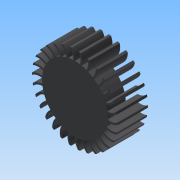
# Autodesk Inventor part: 4020
Saved by Autodesk Inventor 2017 (Build 210142000, 142)
## iProperties
Part Number: 4020
Material: Типовые
Document SubType Name: Modeling
Designer: Max
Mass: 5.03449 g
Surface Area: 54.2386 cm^2
Volume: 5.03449 cm^3
Density: 1 g/cm^3
Appearance: Серый
Author: Max
Autodesk Inventor part; units mm, degrees
ref_plane "YZ Plane" through (0, 0, 0) normal (1, 0, 0) x (0, 1, 0)
ref_plane "XZ Plane" through (0, 0, 0) normal (0, 1, 0) x (-1, 0, 0)
ref_plane "XY Plane" through (0, 0, 0) normal (0, 0, 1) x (1, 0, 0)
sketch "Эскиз1" plane through (0, 0, 0) normal (0, 1, 0) x (-1, 0, 0)
  line L0 (0, 0) -> (0, 30)
  line L1 (0, 30) -> (20.3, 30)
  line L2 (-62.0243, 51.3971) -> (67.3361, 51.3971) construction
  line L3 (67.3361, 51.3971) -> (67.3361, -36.2164) construction
  line L4 (67.3361, -36.2164) -> (-62.0243, -36.2164) construction
  line L5 (-62.0243, -36.2164) -> (-62.0243, 51.3971) construction
  line L6 (20.3, 30) -> (20.3, -25.8683) construction
  line L7 (0, 8.5) -> (47.9124, 8.5) construction
  line L8 (20.3, 30) -> (64.5237, 30) construction
  circle A0 centre (37.8, 27.3) radius 3
  circle A1 centre (37.8, 27.3) radius 1.75
  line L9 (37.8, 27.3) -> (37.8, -7.8) construction
  circle A2 centre (37.8, -7.8) radius 1.75
  circle A3 centre (37.8, -7.8) radius 3
  line L10 (37.8, -7.8) -> (2.8, -7.8) construction
  circle A4 centre (2.8, -7.8) radius 1.75
  circle A5 centre (2.8, -7.8) radius 3
  line L11 (2.8, -7.8) -> (37.8, 27.3) construction
  line L12 (0, 30) -> (40.5, 30) construction
  line L13 (40.5, 30) -> (40.5, -10.5) construction
  line L14 (40.5, -10.5) -> (0, -10.5) construction
  line L15 (0, -10.5) -> (0, 30) construction
  line L16 (0, 0) -> (10.5411, -7.8)
  arc A6 (10.5411, -7.8) -> (30.3802, -7.8) centre (20.4606, 9.7079) ccw
  arc A7 (30.3802, -7.8) -> (40.5, 8.5) centre (20.5113, 9.6185) ccw
  arc A8 (40.5, 8.5) -> (20.3, 30) centre (20.315, 9.7748) ccw
  arc A9 (1.0609, -4.676) -> (0, 0) centre (-2.1861, -2.9543) ccw
  line L17 (0.1496, -6.3946) -> (1.0609, -4.676)
  line L18 (4.7164, -10.1081) -> (7.2118, -8.0362)
  arc A10 (10.5411, -7.8) -> (7.2118, -8.0362) centre (9.0411, -10.2394) ccw
  arc A11 (35.6753, -9.9179) -> (30.3802, -7.8) centre (30.5679, -15.009) ccw
  arc A12 (38.0693, 0) -> (39.868, -5.6267) centre (44.1082, -1.1704) ccw
  arc A13 (29.7654, 27.6564) -> (35.6321, 29.3737) centre (31.2088, 33.6047) ccw
  arc A14 (39.8419, 25.1021) -> (38.1561, 19.3013) centre (43.8447, 20.7935) ccw
  circle A15 centre (20.3, 8.5) radius 14
  arc A16 (30.1091, -7.3215) -> (39.951, 8.5327) centre (20.5113, 9.6185) ccw
  arc A17 (39.951, 8.5327) -> (20.315, 29.45) centre (20.315, 9.7748) ccw
  line L19 (20.315, 29.45) -> (0, 29.45)
  arc A18 (10.8122, -7.3215) -> (30.1091, -7.3215) centre (20.4606, 9.7079) ccw
  line L20 (10.8122, -7.3215) -> (3.3428, 1.6745)
  line L21 (3.3428, 1.6745) -> (0, 1.5217)
  line L22 (0, 1.5217) -> (0, 0)
  line L23 (0, 29.45) -> (0, 30)
  line L24 (0, 29.45) -> (0, 30)
  circle A19 centre (20.3, 8.5) radius 11.5
  circle A20 centre (20.3, 8.5) radius 17
  dimension "d0" = 30
  dimension "d1" = 20.3
  dimension "d2" = 3.5
  dimension "d3" = 17.5
  dimension "d4" = 18.8
  dimension "d5" = 3.5
  dimension "d6" = 16.3
  dimension "d7" = 17.5
  dimension "d8" = 17.5
  dimension "d9" = 3.5
  dimension "d10" = 40.5
  dimension "d11" = 40.5
  dimension "d12" = 21.5
  dimension "d13" = 6
  dimension "d14" = 6
  dimension "d15" = 6
  dimension "d16" = 126.5
  dimension "d17" = 20.2252
  dimension "d18" = 20.0199
  dimension "d19" = 20.1228
  dimension "d20" = 3.6082
  dimension "d21" = 7.2115
  dimension "d22" = 2.8637
  dimension "d23" = 39.703
  dimension "d24" = 0.9113
  dimension "d25" = 6.1513
  dimension "d26" = 5.881
  dimension "d27" = 6.121
  dimension "d28" = 5.8008
  dimension "d29" = 5.8667
  dimension "d30" = 28
  dimension "d31" = 0.55
  dimension "d32" = 0.55
  dimension "d35" = 23
  dimension "d36" = 34
  constraints: 42 end point, 33 point on circle, 21 centre point, 10 tangent, 9 point on line, 7 coincident, 3 collinear, 3 horizontal, 3 perpendicular, 3 vertical, 2 parallel, 3 other
  measures "d0" distance of L0.start L0.end
  measures "d1" distance of L0.end L1.end
  measures "d2" diameter of A1
  measures "d3" distance from line of A0.centre L6
  measures "d4" distance from line of L7 A0.centre
  measures "d5" diameter of A2
  measures "d6" distance from line of L9.end L7
  measures "d7" distance from line of L9.end L6
  measures "d8" distance from line of L6 L10.end
  measures "d9" diameter of A4
  measures "d10" distance of L13.end L14.end
  measures "d11" distance of L12.end L13.end
  measures "d12" distance between parallel lines of L7 L8
  measures "d13" diameter of A0
  measures "d14" diameter of A3
  measures "d15" diameter of A5
  measures "d16" angle of L15 L16
  measures "d17" radius of A8
  measures "d18" radius of A7
  measures "d19" radius of A6
  measures "d20" distance from line of L13 A12.centre
  measures "d21" radius of A11
  measures "d22" radius of A10
  measures "d23" angle of L14 L18
  measures "d24" horizontal distance of L17.start L17.end
  measures "d25" radius of A12
  measures "d26" radius of A14
  measures "d27" radius of A13
  measures "d28" vertical distance of A14.end A0.end
  measures "d29" horizontal distance of A0.start A13.start
  measures "d30" diameter of A15
  measures "d31" radial gap between concentric circles of A7 A16
  measures "d32" radial gap between concentric circles of A6 A18
  measures "d35" diameter of A19
  measures "d36" diameter of A20
extrude "Выдавливание1" add sketch "Эскиз1" along normal blind 12 contours A15 | A19 | A20
sketch "Эскиз2" plane through (-20.3, 12, 8.5) normal (0, 1, 0) x (1, 0, 0)
  circle A0 centre (0, 0) radius 11.5
  circle A1 centre (0, 0) radius 13
  circle A2 centre (0, 0) radius 17 projected
  arc A3 (1.2, 16.9576) -> (0, 13) centre (5.6832, 13.4375) ccw
  arc A4 (2.0528, 16.8756) -> (0.7041, 12.9809) centre (5.6832, 13.4375) ccw
  line L0 (0, 0) -> (0, 22.7332) construction
  point P0 (20.3, 8.5)
  dimension "d40" = 23
  dimension "d41" = 26
  dimension "d42" = 0.7
  dimension "d43" = 1.2
  dimension "d44" = 5
  constraints: 8 point on circle, 4 centre point, 3 coincident, 2 end point, 1 point on line, 1 vertical
  measures "d40" diameter of A0
  measures "d41" diameter of A1
  measures "d42" radial gap between concentric circles of A4 A3
  measures "d43" distance from line of L0 A2.start
  measures "d44" radius of A4
extrude "Выдавливание2" cut sketch "Эскиз2" against normal blind 12 contours A1 A4 A2 A3 | A1 A3 A2 A4
extrude "Выдавливание3" add sketch "Эскиз2" against normal blind 12 contours A1 A3 A2 A4 picked at (0.2619, 13.8155)
pattern_circular "Круговой массив2" count 30 over 360 about axis through (-20.3, 12, 8.5) along (0, -1, 0) of "Выдавливание3"
sketch "Эскиз3" plane through (0, 12, 0) normal (0, 1, 0) x (1, 0, 0)
  arc A0 (-20.3, 4.5) -> (-22.3102, 4.3436) centre (-20.3, -8.5) ccw projected
  arc A1 (-21.8007, 8.4336) -> (-22.3102, 4.3436) centre (-17.5348, 5.8255) ccw projected
  arc A2 (-21.8007, 8.4336) -> (-22.6519, 8.3365) centre (-20.3, -8.5) ccw projected
  arc A3 (-22.6519, 8.3365) -> (-23.0029, 4.2159) centre (-17.5348, 5.8255) ccw projected
  arc A4 (-23.0029, 4.2159) -> (-24.9366, 3.645) centre (-20.3, -8.5) ccw projected
  arc A5 (-25.2886, 7.7516) -> (-24.9366, 3.645) centre (-20.5737, 6.0873) ccw projected
  arc A6 (-25.2886, 7.7516) -> (-26.101, 7.4796) centre (-20.3, -8.5) ccw projected
  arc A7 (-26.101, 7.4796) -> (-25.5876, 3.3761) centre (-20.5737, 6.0873) ccw projected
  arc A8 (-25.5876, 3.3761) -> (-27.3604, 2.4156) centre (-20.3, -8.5) ccw projected
  arc A9 (-28.5585, 6.3593) -> (-27.3604, 2.4156) centre (-23.6006, 5.7117) ccw projected
  arc A10 (-28.5585, 6.3593) -> (-29.2966, 5.9243) centre (-20.3, -8.5) ccw projected
  arc A11 (-29.2966, 5.9243) -> (-27.9412, 2.0172) centre (-23.6006, 5.7117) ccw projected
  arc A12 (-27.9412, 2.0172) -> (-29.4756, 0.7092) centre (-20.3, -8.5) ccw projected
  arc A13 (-31.4674, 4.3175) -> (-29.4756, 0.7092) centre (-26.4832, 4.7149) ccw projected
  arc A14 (-31.4674, 4.3175) -> (-32.099, 3.7386) centre (-20.3, -8.5) ccw projected
  arc A15 (-32.099, 3.7386) -> (-29.9609, 0.1987) centre (-26.4832, 4.7149) ccw projected
  arc A16 (-29.9609, 0.1987) -> (-31.1898, -1.3998) centre (-20.3, -8.5) ccw projected
  arc A17 (-33.8883, 1.7156) -> (-31.1898, -1.3998) centre (-29.0956, 3.1405) ccw projected
  arc A18 (-33.8883, 1.7156) -> (-34.3857, 1.018) centre (-20.3, -8.5) ccw projected
  arc A19 (-34.3857, 1.018) -> (-31.5583, -2) centre (-29.0956, 3.1405) ccw projected
  arc A20 (-31.5583, -2) -> (-32.428, -3.8191) centre (-20.3, -8.5) ccw projected
  arc A21 (-35.7153, -1.3328) -> (-32.428, -3.8191) centre (-31.3236, 1.0574) ccw projected
  arc A22 (-35.7153, -1.3328) -> (-36.0568, -2.1185) centre (-20.3, -8.5) ccw projected
  arc A23 (-36.0568, -2.1185) -> (-32.6637, -4.4828) centre (-31.3236, 1.0574) ccw projected
  arc A24 (-32.6637, -4.4828) -> (-33.1362, -6.4429) centre (-20.3, -8.5) ccw projected
  arc A25 (-36.8686, -4.6944) -> (-33.1362, -6.4429) centre (-33.0698, -1.4433) ccw projected
  arc A26 (-36.8686, -4.6944) -> (-37.0393, -5.534) centre (-20.3, -8.5) ccw projected
  arc A27 (-37.0393, -5.534) -> (-33.2288, -7.1411) centre (-33.0698, -1.4433) ccw projected
  arc A28 (-33.2288, -7.1411) -> (-33.2834, -9.1567) centre (-20.3, -8.5) ccw projected
  arc A29 (-37.2977, -8.2224) -> (-33.2834, -9.1567) centre (-34.2579, -4.2525) ccw projected
  arc A30 (-37.2977, -8.2224) -> (-37.2901, -9.0791) centre (-20.3, -8.5) ccw projected
  arc A31 (-37.2901, -9.0791) -> (-33.2288, -9.8589) centre (-34.2579, -4.2525) ccw projected
  arc A32 (-33.2288, -9.8589) -> (-32.8632, -11.8417) centre (-20.3, -8.5) ccw projected
  arc A33 (-36.984, -11.7625) -> (-32.8632, -11.8417) centre (-34.836, -7.2474) ccw projected
  arc A34 (-36.984, -11.7625) -> (-36.7985, -12.5989) centre (-20.3, -8.5) ccw projected
  arc A35 (-36.7985, -12.5989) -> (-32.6637, -12.5172) centre (-34.836, -7.2474) ccw projected
  arc A36 (-32.6637, -12.5172) -> (-31.8938, -14.3807) centre (-20.3, -8.5) ccw projected
  arc A37 (-35.9411, -15.16) -> (-31.8938, -14.3807) centre (-34.7788, -10.297) ccw projected
  arc A38 (-35.9411, -15.16) -> (-35.5857, -15.9396) centre (-20.3, -8.5) ccw projected
  arc A39 (-35.5857, -15.9396) -> (-31.5583, -15) centre (-34.7788, -10.297) ccw projected
  arc A40 (-31.5583, -15) -> (-30.4178, -16.6627) centre (-20.3, -8.5) ccw projected
  arc A41 (-34.2146, -18.2664) -> (-30.4178, -16.6627) centre (-34.0888, -13.268) ccw projected
  arc A42 (-34.2146, -18.2664) -> (-33.7049, -18.9551) centre (-20.3, -8.5) ccw projected
  arc A43 (-33.7049, -18.9551) -> (-29.9609, -17.1987) centre (-34.0888, -13.268) ccw projected
  arc A44 (-29.9609, -17.1987) -> (-28.4996, -18.5879) centre (-20.3, -8.5) ccw projected
  arc A45 (-31.88, -20.946) -> (-28.4996, -18.5879) centre (-32.7962, -16.0307) ccw projected
  arc A46 (-31.88, -20.946) -> (-31.2382, -21.5136) centre (-20.3, -8.5) ccw projected
  arc A47 (-31.2382, -21.5136) -> (-27.9412, -19.0172) centre (-32.7962, -16.0307) ccw projected
  arc A48 (-27.9412, -19.0172) -> (-26.223, -20.0723) centre (-20.3, -8.5) ccw projected
  arc A49 (-29.0393, -23.0817) -> (-26.223, -20.0723) centre (-30.9574, -18.4642) ccw projected
  arc A50 (-29.0393, -23.0817) -> (-28.2935, -23.5034) centre (-20.3, -8.5) ccw projected
  arc A51 (-28.2935, -23.5034) -> (-25.5876, -20.3761) centre (-30.9574, -18.4642) ccw projected
  arc A52 (-25.5876, -20.3761) -> (-23.6876, -21.0509) centre (-20.3, -8.5) ccw projected
  arc A53 (-25.8166, -24.58) -> (-23.6876, -21.0509) centre (-28.6528, -20.4623) ccw projected
  arc A54 (-25.8166, -24.58) -> (-24.9995, -24.8375) centre (-20.3, -8.5) ccw projected
  arc A55 (-24.9995, -24.8375) -> (-23.0029, -21.2159) centre (-28.6528, -20.4623) ccw projected
  arc A56 (-23.0029, -21.2159) -> (-21.0041, -21.4809) centre (-20.3, -8.5) ccw projected
  arc A57 (-22.3528, -25.3756) -> (-21.0041, -21.4809) centre (-25.9832, -21.9375) ccw projected
  arc A58 (-22.3528, -25.3756) -> (-21.5, -25.4576) centre (-20.3, -8.5) ccw projected
  arc A59 (-21.5, -25.4576) -> (-20.3, -21.5) centre (-25.9832, -21.9375) ccw projected
  arc A60 (-20.3, -21.5) -> (-18.2898, -21.3436) centre (-20.3, -8.5) ccw projected
  arc A61 (-18.7993, -25.4336) -> (-18.2898, -21.3436) centre (-23.0652, -22.8255) ccw projected
  arc A62 (-18.7993, -25.4336) -> (-17.9481, -25.3365) centre (-20.3, -8.5) ccw projected
  arc A63 (-17.9481, -25.3365) -> (-17.5971, -21.2159) centre (-23.0652, -22.8255) ccw projected
  arc A64 (-17.5971, -21.2159) -> (-15.6634, -20.645) centre (-20.3, -8.5) ccw projected
  arc A65 (-15.3114, -24.7516) -> (-15.6634, -20.645) centre (-20.0263, -23.0873) ccw projected
  arc A66 (-15.3114, -24.7516) -> (-14.499, -24.4796) centre (-20.3, -8.5) ccw projected
  arc A67 (-14.499, -24.4796) -> (-15.0124, -20.3761) centre (-20.0263, -23.0873) ccw projected
  arc A68 (-15.0124, -20.3761) -> (-13.2396, -19.4156) centre (-20.3, -8.5) ccw projected
  arc A69 (-12.0415, -23.3593) -> (-13.2396, -19.4156) centre (-16.9994, -22.7117) ccw projected
  arc A70 (-12.0415, -23.3593) -> (-11.3034, -22.9243) centre (-20.3, -8.5) ccw projected
  arc A71 (-11.3034, -22.9243) -> (-12.6588, -19.0172) centre (-16.9994, -22.7117) ccw projected
  arc A72 (-12.6588, -19.0172) -> (-11.1244, -17.7092) centre (-20.3, -8.5) ccw projected
  arc A73 (-9.1326, -21.3175) -> (-11.1244, -17.7092) centre (-14.1168, -21.7149) ccw projected
  arc A74 (-9.1326, -21.3175) -> (-8.501, -20.7386) centre (-20.3, -8.5) ccw projected
  arc A75 (-8.501, -20.7386) -> (-10.6391, -17.1987) centre (-14.1168, -21.7149) ccw projected
  arc A76 (-10.6391, -17.1987) -> (-9.4102, -15.6002) centre (-20.3, -8.5) ccw projected
  arc A77 (-6.7117, -18.7156) -> (-9.4102, -15.6002) centre (-11.5044, -20.1405) ccw projected
  arc A78 (-6.7117, -18.7156) -> (-6.2143, -18.018) centre (-20.3, -8.5) ccw projected
  arc A79 (-6.2143, -18.018) -> (-9.0417, -15) centre (-11.5044, -20.1405) ccw projected
  arc A80 (-9.0417, -15) -> (-8.172, -13.1809) centre (-20.3, -8.5) ccw projected
  arc A81 (-4.8847, -15.6672) -> (-8.172, -13.1809) centre (-9.2764, -18.0574) ccw projected
  arc A82 (-4.8847, -15.6672) -> (-4.5432, -14.8815) centre (-20.3, -8.5) ccw projected
  arc A83 (-4.5432, -14.8815) -> (-7.9363, -12.5172) centre (-9.2764, -18.0574) ccw projected
  arc A84 (-7.9363, -12.5172) -> (-7.4638, -10.5571) centre (-20.3, -8.5) ccw projected
  arc A85 (-3.7314, -12.3056) -> (-7.4638, -10.5571) centre (-7.5302, -15.5567) ccw projected
  arc A86 (-3.7314, -12.3056) -> (-3.5607, -11.466) centre (-20.3, -8.5) ccw projected
  arc A87 (-3.5607, -11.466) -> (-7.3712, -9.8589) centre (-7.5302, -15.5567) ccw projected
  arc A88 (-7.3712, -9.8589) -> (-7.3166, -7.8433) centre (-20.3, -8.5) ccw projected
  arc A89 (-3.3023, -8.7776) -> (-7.3166, -7.8433) centre (-6.3421, -12.7475) ccw projected
  arc A90 (-3.3023, -8.7776) -> (-3.3099, -7.9209) centre (-20.3, -8.5) ccw projected
  arc A91 (-3.3099, -7.9209) -> (-7.3712, -7.1411) centre (-6.3421, -12.7475) ccw projected
  arc A92 (-7.3712, -7.1411) -> (-7.7368, -5.1583) centre (-20.3, -8.5) ccw projected
  arc A93 (-3.616, -5.2375) -> (-7.7368, -5.1583) centre (-5.764, -9.7526) ccw projected
  arc A94 (-3.616, -5.2375) -> (-3.8015, -4.4011) centre (-20.3, -8.5) ccw projected
  arc A95 (-3.8015, -4.4011) -> (-7.9363, -4.4828) centre (-5.764, -9.7526) ccw projected
  arc A96 (-7.9363, -4.4828) -> (-8.7062, -2.6193) centre (-20.3, -8.5) ccw projected
  arc A97 (-4.6589, -1.84) -> (-8.7062, -2.6193) centre (-5.8212, -6.703) ccw projected
  arc A98 (-4.6589, -1.84) -> (-5.0143, -1.0604) centre (-20.3, -8.5) ccw projected
  arc A99 (-5.0143, -1.0604) -> (-9.0417, -2) centre (-5.8212, -6.703) ccw projected
  arc A100 (-9.0417, -2) -> (-10.1822, -0.3373) centre (-20.3, -8.5) ccw projected
  arc A101 (-6.3854, 1.2664) -> (-10.1822, -0.3373) centre (-6.5112, -3.732) ccw projected
  arc A102 (-6.3854, 1.2664) -> (-6.8951, 1.9551) centre (-20.3, -8.5) ccw projected
  arc A103 (-6.8951, 1.9551) -> (-10.6391, 0.1987) centre (-6.5112, -3.732) ccw projected
  arc A104 (-10.6391, 0.1987) -> (-12.1004, 1.5879) centre (-20.3, -8.5) ccw projected
  arc A105 (-8.72, 3.946) -> (-12.1004, 1.5879) centre (-7.8038, -0.9693) ccw projected
  arc A106 (-8.72, 3.946) -> (-9.3618, 4.5136) centre (-20.3, -8.5) ccw projected
  arc A107 (-9.3618, 4.5136) -> (-12.6588, 2.0172) centre (-7.8038, -0.9693) ccw projected
  arc A108 (-12.6588, 2.0172) -> (-14.377, 3.0723) centre (-20.3, -8.5) ccw projected
  arc A109 (-11.5607, 6.0817) -> (-14.377, 3.0723) centre (-9.6426, 1.4642) ccw projected
  arc A110 (-11.5607, 6.0817) -> (-12.3065, 6.5034) centre (-20.3, -8.5) ccw projected
  arc A111 (-12.3065, 6.5034) -> (-15.0124, 3.3761) centre (-9.6426, 1.4642) ccw projected
  arc A112 (-15.0124, 3.3761) -> (-16.9124, 4.0509) centre (-20.3, -8.5) ccw projected
  arc A113 (-14.7834, 7.58) -> (-16.9124, 4.0509) centre (-11.9472, 3.4623) ccw projected
  arc A114 (-14.7834, 7.58) -> (-15.6005, 7.8375) centre (-20.3, -8.5) ccw projected
  arc A115 (-15.6005, 7.8375) -> (-17.5971, 4.2159) centre (-11.9472, 3.4623) ccw projected
  arc A116 (-17.5971, 4.2159) -> (-19.5959, 4.4809) centre (-20.3, -8.5) ccw projected
  arc A117 (-18.2472, 8.3756) -> (-19.5959, 4.4809) centre (-14.6168, 4.9375) ccw projected
  arc A118 (-18.2472, 8.3756) -> (-19.1, 8.4576) centre (-20.3, -8.5) ccw projected
  arc A119 (-19.1, 8.4576) -> (-20.3, 4.5) centre (-14.6168, 4.9375) ccw projected
  arc A120 (-29.2966, 5.9243) -> (-27.9412, 2.0172) centre (-23.6006, 5.7117) ccw projected
  circle A121 centre (-20.3, -8.5) radius 17
  circle A122 centre (-20.3, -8.5) radius 13
  circle A123 centre (-20.3, -8.5) radius 11.5
  point P0 (0, 0)
  dimension "d55" = 23
  constraints: 3 coincident, 2 centre point, 3 other
  measures "d55" diameter of A123
extrude "Выдавливание4" cut sketch "Эскиз3" against normal blind 10 contours A122 A116 A112 A108 A104 A100 A96 A92 A88 A84 A80 A76 A72 A68 A64 A60 A56 A52 A48 A44 A40 A36 A32 A28 A24 A20 A16 A12 A8 A4 A0
extrude "Выдавливание5" cut sketch "Эскиз3" against normal blind 3 contours A123
fillet "Сопряжение1" radius 0.5 1 edges at (-31.8, 9, 8.5)
